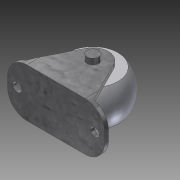
# Autodesk Inventor part: rolka_meblowa_32mm
Saved by Autodesk Inventor 2013 (Build 170138000, 138)
## iProperties
Created: 2014-04-27
Part Number: rolka_meblowa_32mm
Material: Generic
Document SubType Name: Modeling
Designer: Masta
Density: 1 g/cm^3
Author: Masta
Autodesk Inventor part; units mm, degrees
ref_plane "YZ Plane" through (0, 0, 0) normal (1, 0, 0) x (0, 1, 0)
ref_plane "XZ Plane" through (0, 0, 0) normal (0, 1, 0) x (-1, 0, 0)
ref_plane "XY Plane" through (0, 0, 0) normal (0, 0, 1) x (1, 0, 0)
sketch "Sketch1" plane through (0, 0, 0) normal (0, 0, 1) x (1, 0, 0)
  line L0 (-25, 0) -> (25, 0)
  line L1 (25, 0) -> (25, 2)
  line L2 (25, 2) -> (-25, 2)
  line L3 (-25, 2) -> (-25, 0)
  line L4 (-17.5, 2) -> (-7.1477, 22.5932)
  line L5 (7.1477, 22.5932) -> (17.5, 2)
  line L6 (0, 19) -> (0, 2) construction
  arc A0 (7.1477, 22.5932) -> (-7.1477, 22.5932) centre (0, 19) ccw
  circle A1 centre (0, 19) radius 3
  point P0 (0, 0)
  point P1 (0, 0)
  dimension "d0" = 50
  dimension "d1" = 2
  dimension "d2" = 35
  dimension "d3" = 19
  dimension "d4" = 8
  dimension "d5" = 6
  constraints: 14 end point, 3 coincident, 2 centre point, 2 midpoint, 2 parallel, 2 point on circle, 2 point on line, 1 horizontal, 1 perpendicular, 1 tangent, 1 other
  measures "d0" distance of L2.end L1.end
  measures "d1" distance of L1.end L0.end
  measures "d2" distance of L5.end L4.start
  measures "d3" distance from line of L0 L6.start
  measures "d4" radius of A0
  measures "d5" diameter of A1
extrude "Extrusion1" add sketch "Sketch1" along normal mid plane 25
extrude "Extrusion3" add sketch "Sketch1" along normal mid plane 31 contours A1
extrude "Extrusion2" cut sketch "Sketch1" along normal mid plane 21 contours L4 A0 L5 L2
sketch "Sketch2" plane through (0, 0, 0) normal (1, 0, 0) x (0, 1, 0)
  line L0 (16, -10.5) -> (16, 10.5) projected
  line L1 (16, 10.5) -> (2, 10.5) projected
  line L2 (2, 10.5) -> (2, -10.5) projected
  line L3 (2, -10.5) -> (16, -10.5) projected
  line L4 (22, -12.5) -> (22, -15.5) projected
  line L5 (22, -15.5) -> (16, -15.5) projected
  line L6 (16, -15.5) -> (16, -12.5) projected
  line L7 (16, -12.5) -> (0, -12.5) projected
  line L8 (0, -12.5) -> (0, 12.5) projected
  line L9 (0, 12.5) -> (16, 12.5) projected
  line L10 (16, 12.5) -> (16, 15.5) projected
  line L11 (16, 15.5) -> (22, 15.5) projected
  line L12 (22, 15.5) -> (22, 12.5) projected
  line L13 (22, 12.5) -> (27, 12.5) projected
  line L14 (27, 12.5) -> (27, 10.5) projected
  line L15 (27, 10.5) -> (22, 10.5) projected
  line L16 (22, 10.5) -> (22, -10.5) projected
  line L17 (22, -10.5) -> (27, -10.5) projected
  line L18 (27, -10.5) -> (27, -12.5) projected
  line L19 (27, -12.5) -> (22, -12.5) projected
  line L20 (19, 15.5) -> (19, -15.5)
  line L21 (23, 9.5) -> (23, -9.5)
  line L22 (23, -9.5) -> (31.8744, -9.5)
  line L23 (23, 9.5) -> (31.8744, 9.5)
  arc A0 (31.8744, -9.5) -> (31.8744, 9.5) centre (19, 0) ccw
  line L24 (19, 0) -> (2, 0) construction
  line L25 (35, 9.5) -> (35, -9.5) construction
  line L26 (31.8744, 9.5) -> (35, 9.5) construction
  line L27 (35, -9.5) -> (31.8744, -9.5) construction
  point P0 (0, 0)
  dimension "d12" = 1
  dimension "d13" = 1
  dimension "d14" = 16
  dimension "d15" = 16
  constraints: 14 end point, 4 perpendicular, 3 parallel, 2 midpoint, 2 point on circle, 1 centre point, 1 symmetric about line, 1 tangent, 1 other
  measures "d12" distance between parallel lines of L15 L23
  measures "d13" distance between parallel lines of L16 L21
  measures "d14" distance between parallel lines of L20 L25
  measures "d15" radius of A0
revolve "Revolution1" add sketch "Sketch2" angle 360 about axis through (0, 19, 15.5) along (0, 0, -1) contours L23 A0 L22 L21
fillet "Fillet1" radius 10 4 edges at (-25, 1, -12.5) (-25, 1, 12.5) (25, 1, 12.5) (25, 1, -12.5)
sketch "Sketch3" plane through (-15, 0, 12.5) normal (0, -1, 0) x (1, 0, 0)
  line L0 (40, -15) -> (40, -10) projected
  line L1 (0, 0) -> (30, 0) projected
  line L2 (-10, -10) -> (-10, -15) projected
  line L3 (30, -25) -> (0, -25) projected
  line L4 (-10, -12.5) -> (40, -12.5) construction
  line L5 (15, 0) -> (15, -25) construction
  point P0 (15, -12.5)
  point P1 (-5, -12.5)
  point P2 (35, -12.5)
  dimension "d18" = 40
  constraints: 4 end point, 4 midpoint, 2 point on line, 1 symmetric about line
  measures "d18" distance of point (35, -12.5) point (-5, -12.5)
hole "Hole1" at (-20, 0, 0) at (20, 0, 0) direction (0, 1, 0) diameter 4.5 end through all
body "Solid1"
